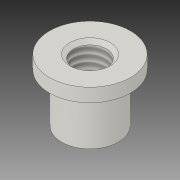
# Autodesk Inventor part: 9775036360R
Saved by Autodesk Inventor 2019.1 (Build 231200000, 200)
## iProperties
Part Number: 9775036360R
Material: Stahl, geschmiedet
Document SubType Name: Modeling
Designer: rYan
Mass: 0.511087 g
Surface Area: 1.68728 cm^2
Volume: 0.0651066 cm^3
Density: 7.85 g/cm^3
Appearance: Stahl
Author: rYan
Autodesk Inventor part; units mm, degrees
ref_plane "YZ Plane" through (0, 0, 0) normal (1, 0, 0) x (0, 1, 0)
ref_plane "XZ Plane" through (0, 0, 0) normal (0, 1, 0) x (-1, 0, 0)
ref_plane "XY Plane" through (0, 0, 0) normal (0, 0, 1) x (1, 0, 0)
sketch "Skizze1" plane through (0, 0, 0) normal (1, 0, 0) x (0, 1, 0)
  line L0 (0, 1) -> (0, -3.6)
  line L1 (0, 1) -> (-3, 1)
  line L2 (-3, 1) -> (-3, 0)
  line L3 (-3, 0) -> (-2.1, 0)
  line L4 (-2.1, 0) -> (-2.1, -3.6)
  line L5 (-2.1, -3.6) -> (0, -3.6)
  point P0 (0, 0)
  dimension "d0" = 6
  dimension "d1" = 4.2
  dimension "d2" = 1
  dimension "Länge" = 3.6
  constraints: 12 end point, 4 perpendicular, 2 point on line, 1 horizontal, 1 vertical
  measures "d0" diameter of L2 L0
  measures "d1" diameter of L4 L0
  measures "d2" distance of L1.end L2.end
  measures "Länge" distance between parallel lines of L5 L3
revolve "Umdrehung1" add sketch "Skizze1" angle 360 about axis through (0, 0, 1) along (0, 0, -1)
sketch "Skizze2" plane through (0, 0, 1) normal (0, 0, 1) x (1, 0, 0)
  point P0 (0, 0)
  point P1 (0, 0)
  constraints: 1 coincident
hole "Bohrung1" at (0, 0, 1) direction (0, 0, -1) diameter 2.459 end through all countersink diameter 3 countersink angle 90 thread size "M3x0.5" class "6H" standard "ISO Metric profile"
